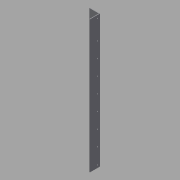
# Autodesk Inventor part: 26in Angle Channel
Saved by Autodesk Inventor 2013 (Build 170138000, 138)
## iProperties
Created: 2013-01-27
Part Number: 26in Angle Channel
Material: Aluminum 6061
Document SubType Name: Modeling
Designer: Naphat
Density: 1 g/cm^3
Author: Naphat
Autodesk Inventor part; units mm, degrees
ref_plane "YZ Plane" through (0, 0, 0) normal (1, 0, 0) x (0, 1, 0)
ref_plane "XZ Plane" through (0, 0, 0) normal (0, 1, 0) x (-1, 0, 0)
ref_plane "XY Plane" through (0, 0, 0) normal (0, 0, 1) x (1, 0, 0)
sketch "Sketch1" plane through (0, 0, 0) normal (0, 1, 0) x (-1, 0, 0)
  line L0 (0, 0) -> (50, 0)
  line L1 (50, 0) -> (50, 3)
  line L2 (0, 0) -> (0, 50)
  line L3 (0, 50) -> (3, 50)
  line L4 (3, 50) -> (3, 3)
  line L5 (3, 3) -> (50, 3)
  dimension "d0" = 50
  dimension "d1" = 3
  dimension "d2" = 50
  dimension "d3" = 3
  constraints: 12 end point, 3 perpendicular, 2 parallel, 1 horizontal
  measures "d0" distance of L0.start L0.end
  measures "d1" distance of L0.end L1.end
  measures "d2" distance of L0.start L2.end
  measures "d3" distance of L2.end L3.end
extrude "Extrusion1" add sketch "Sketch1" along normal blind 660.4
sketch "Sketch2" plane through (-3, 0, 3) normal (-1, 0, 0) x (0, 0, 1)
  line L0 (0, 0) -> (47, 0) projected
  line L1 (-3, 0) -> (-3, 660.4) projected
  line L2 (-3, 13.8784) -> (9.7, 13.8784) construction
  line L3 (9.7, 0) -> (9.7, 15.7) construction
  line L4 (9.7, 0) -> (25.4, 0) construction
  line L5 (9.7, 15.7) -> (9.7, 91.9) construction
  line L6 (9.7, 91.9) -> (9.7, 168.1) construction
  line L7 (9.7, 168.1) -> (9.7, 244.3) construction
  line L8 (9.7, 244.3) -> (9.7, 320.5) construction
  line L9 (9.7, 320.5) -> (9.7, 396.7) construction
  line L10 (9.7, 396.7) -> (9.7, 472.9) construction
  line L11 (9.7, 472.9) -> (9.7, 549.1) construction
  line L12 (0, 660.4) -> (47, 660.4) construction
  line L13 (9.7, 661.3513) -> (9.7, 645.6513) construction
  line L14 (9.7, 549.1) -> (9.7, 625.3) construction
  circle A0 centre (9.7, 645.6513) radius 3.175
  circle A1 centre (9.7, 549.1) radius 3.175
  circle A2 centre (9.7, 472.9) radius 3.175
  circle A3 centre (9.7, 396.7) radius 3.175
  circle A4 centre (9.7, 320.5) radius 3.175
  circle A5 centre (9.7, 244.3) radius 3.175
  circle A6 centre (9.7, 168.1) radius 3.175
  circle A7 centre (9.7, 91.9) radius 3.175
  circle A8 centre (9.7, 13.8784) radius 3.175
  dimension "d26" = 12.7
  dimension "d28" = 15.7
  dimension "d29" = 90
  dimension "d30" = 76.2
  dimension "d31" = 180
  dimension "d32" = 76.2
  dimension "d33" = 180
  dimension "d34" = 76.2
  dimension "d35" = 180
  dimension "d36" = 76.2
  dimension "d37" = 180
  dimension "d38" = 76.2
  dimension "d39" = 180
  dimension "d40" = 76.2
  dimension "d41" = 180
  dimension "d42" = 76.2
  dimension "d43" = 180
  dimension "d44" = 15.7
  dimension "d45" = 76.2
  dimension "d46" = 6.35
  dimension "d47" = 6.35
  dimension "d48" = 6.35
  dimension "d49" = 6.35
  dimension "d50" = 6.35
  dimension "d51" = 6.35
  dimension "d52" = 6.35
  dimension "d53" = 6.35
  dimension "d54" = 6.35
  constraints: 24 end point, 9 centre point, 9 coincident, 8 collinear, 4 perpendicular, 2 point on line, 1 horizontal
  measures "d26" distance of L2.start L2.end
  measures "d28" distance of L3.start L3.end
  measures "d29" angle of L4 L3
  measures "d30" distance of L3.end L5.end
  measures "d31" angle of L5 L3
  measures "d32" distance of L5.end L6.end
  measures "d33" angle of L6 L5
  measures "d34" distance of L6.end L7.end
  measures "d35" angle of L7 L6
  measures "d36" distance of L7.end L8.end
  measures "d37" angle of L8 L7
  measures "d38" distance of L8.end L9.end
  measures "d39" angle of L9 L8
  measures "d40" distance of L9.end L10.end
  measures "d41" angle of L10 L9
  measures "d42" distance of L10.end L11.end
  measures "d43" angle of L11 L10
  measures "d44" distance of L13.start L13.end
  measures "d45" distance of L11.end L14.end
  measures "d46" diameter of A0
  measures "d47" diameter of A1
  measures "d48" diameter of A2
  measures "d49" diameter of A3
  measures "d50" diameter of A4
  measures "d51" diameter of A5
  measures "d52" diameter of A6
  measures "d53" diameter of A7
  measures "d54" diameter of A8
extrude "Extrusion2" cut sketch "Sketch2" against normal blind 25.4
body "Solid1"
